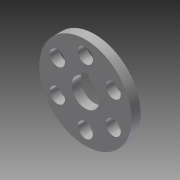
# Autodesk Inventor part: Hub for rachet
Saved by Autodesk Inventor 2013 (Build 170138000, 138)
## iProperties
Created: 2013-02-04
Part Number: Hub for rachet
Material: Steel
Document SubType Name: Modeling
Designer: Arpan
Density: 7.85 g/cm^3
Mass: 39.4696 g
Surface Area: 40.4738 cm^2
Volume: 5.02798 cm^3
Author: Arpan
Autodesk Inventor part; units mm, degrees
ref_plane "YZ Plane" through (0, 0, 0) normal (1, 0, 0) x (0, 1, 0)
ref_plane "XZ Plane" through (0, 0, 0) normal (0, 1, 0) x (-1, 0, 0)
ref_plane "XY Plane" through (0, 0, 0) normal (0, 0, 1) x (1, 0, 0)
sketch "Sketch1" plane through (0, 0, 0) normal (0, 0, 1) x (1, 0, 0)
  arc A0 (-1.1906, 4.6113) -> (1.1906, 4.6113) centre (0, 0) ccw
  circle A1 centre (0, 0) radius 15.875
  line L0 (0, 4.7625) -> (0, 11.1125)
  circle A2 centre (0, 11.1125) radius 2.5908
  circle A3 centre (-9.6237, 5.5563) radius 2.5908
  circle A4 centre (-9.6237, -5.5562) radius 2.5908
  circle A5 centre (0, -11.1125) radius 2.5908
  circle A6 centre (9.6237, -5.5563) radius 2.5908
  circle A7 centre (9.6237, 5.5562) radius 2.5908
  line L1 (0, 0) -> (-1.1906, 0)
  line L2 (0, 0) -> (1.1906, 0)
  line L3 (1.1906, 0) -> (1.1906, 4.6113)
  line L4 (1.1906, 4.6113) -> (1.1906, 5.8019)
  line L5 (1.1906, 5.8019) -> (-1.1906, 5.8019)
  line L6 (-1.1906, 5.8019) -> (-1.1906, 4.6113)
  dimension "d0" = 9.525
  dimension "d1" = 31.75
  dimension "d2" = 6.35
  dimension "d3" = 5.1816
  dimension "d6" = 360
  dimension "d10" = 1.1906
  dimension "d11" = 1.1906
  dimension "d12" = 1.1906
  constraints: 14 end point, 8 centre point, 3 coincident, 3 perpendicular, 2 collinear, 2 point on circle, 1 vertical, 13 other
  measures "d0" diameter of A0
  measures "d1" diameter of A1
  measures "d2" distance of L0.start L0.end
  measures "d3" diameter of A2
  measures "d10" distance of L1.start L1.end
  measures "d11" distance of L1.start L2.end
  measures "d12" distance of L3.end L4.end
extrude "Extrusion1" add sketch "Sketch1" along normal blind 3.175
body "Solid1"
